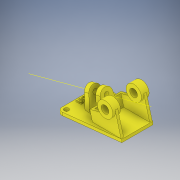
# Autodesk Inventor part: Piesa 1
Saved by Autodesk Inventor 2019.4 (Build 234330000, 330)
## iProperties
Created: 2020-02-23
Part Number: Piesa 1
Material: Steel, Carbon
Document SubType Name: Modeling
Designer: Gabriel
Density: 7.85 g/cm^3
Appearance: Canary
Author: Gabriel
Autodesk Inventor part; units mm, degrees
ref_plane "YZ Plane" through (0, 0, 0) normal (1, 0, 0) x (0, 1, 0)
ref_plane "XZ Plane" through (0, 0, 0) normal (0, 1, 0) x (-1, 0, 0)
ref_plane "XY Plane" through (0, 0, 0) normal (0, 0, 1) x (1, 0, 0)
sketch "Sketch1" plane through (0, 0, 0) normal (0, 0, 1) x (1, 0, 0)
  line L0 (-28.987733, 0) -> (173.926398, 0)
  line L1 (176.623272, 47.326063) -> (-29.437212, -7.887677)
  line L2 (101.214161, 39.543567) -> (109.907493, 41.872938)
  line L3 (109.907493, 41.872938) -> (118.96616, 8.065534)
  line L4 (118.96616, 8.065534) -> (132.489121, 11.689001)
  line L5 (132.489121, 11.689001) -> (123.430455, 45.496405)
  line L6 (123.430455, 45.496405) -> (132.123787, 47.825776)
  line L7 (132.123787, 47.825776) -> (144.938665, 0)
  line L8 (144.938665, 0) -> (111.809827, 0)
  line L9 (111.809827, 0) -> (101.214161, 39.543567)
  point P0 (0, 0)
  dimension "d0" = 9
  dimension "d1" = 14
  dimension "d2" = 9
  dimension "d3" = 35
  dimension "d4" = 117
  dimension "d5" = 12
  constraints: 16 end point, 6 perpendicular, 1 collinear, 1 horizontal, 1 point on line
  measures "d0" distance of L2.start L2.end
  measures "d1" distance of L3.end L4.end
  measures "d2" distance of L5.end L6.end
  measures "d3" distance between parallel lines of L2 L4
  measures "d4" distance from line of point (0, 0) L3
  measures "d5" distance between parallel lines of L6 L1
extrude "Extrusion1" add sketch "Sketch1" along normal mid plane 50 contours L9 L1 L3 L4 L5 L7 L0 | L9 L2 L3 L1 | L1 L5 L6 L7
sketch "Sketch2" plane through (111.809827, 0, -25) normal (-0.9659258, -0.258819, 0) x (0, 0, 1)
  line L0 (25, 64.840128) -> (25, -46.47118)
  line L1 (50, -8.574374) -> (0, -8.574374)
  line L2 (0, 40.938513) -> (50, 40.938513)
  line L3 (1.569954, -23.574374) -> (48.430046, -23.574374)
  line L4 (48.430046, -23.574374) -> (36.737771, 31.433453)
  line L5 (1.569954, -23.574374) -> (13.262229, 31.433453)
  arc A0 (36.737771, 31.433453) -> (13.262229, 31.433453) centre (25, 28.938513) ccw
  point P0 (25, 28.938513)
  point P1 (25, 40.938513)
  dimension "d8" = 15
  dimension "d9" = 12
  dimension "d10" = 78
  dimension "d11" = 78
  constraints: 6 end point, 3 point on circle, 2 tangent, 1 centre point, 1 horizontal, 1 midpoint
  measures "d8" distance between parallel lines of L1 L3
  measures "d9" radius of A0
  measures "d10" angle of L5 L3
  measures "d11" angle of L3 L4
extrude "Extrusion2" cut sketch "Sketch2" against normal through all keep common part
sketch "Sketch3" plane through (0, 0, 0) normal (0, 0, 1) x (1, 0, 0)
  line L0 (176.623272, 47.326063) -> (-29.437212, -7.887677)
  line L1 (-28.987733, 0) -> (173.926398, 0)
  line L2 (132.98317, 25.3) -> (156.16539, 31.511657)
  line L3 (156.16539, 31.511657) -> (153.582206, 41.152228)
  line L4 (182.559981, 48.9168) -> (195.667198, 0)
  line L5 (195.667198, 0) -> (139.762284, 0)
  line L6 (132.98317, 25.3) -> (139.762284, 0)
  point P0 (0, 0)
  point P1 (144.938665, 0)
  dimension "d14" = 24
  dimension "d15" = 30
  dimension "d16" = 49
  dimension "d17" = 5
  dimension "d18" = 25.3
  constraints: 10 end point, 4 point on line, 2 perpendicular, 1 parallel
  measures "d14" distance of L2.start L2.end
  measures "d15" distance between parallel lines of L4 L3
  measures "d16" distance from line of point (144.939, 0) L4
  measures "d17" distance from line of point (144.939, 0) L6
  measures "d18" distance from line of L1 L2.start
sketch "Sketch3 outline for Extrusion3" plane through (0, 0, 0) normal (0, 0, 1) x (1, 0, 0)
  line L0 (156.16539, 31.511657) -> (132.98317, 25.3)
  line L1 (153.582206, 41.152228) -> (156.16539, 31.511657)
  line L2 (182.559981, 48.9168) -> (153.582206, 41.152228)
  line L3 (195.667198, 0) -> (182.559981, 48.9168)
  line L4 (139.762284, 0) -> (195.667198, 0)
  line L5 (132.98317, 25.3) -> (139.762284, 0)
extrude "Extrusion3" add sketch "Sketch3 outline for Extrusion3" along normal mid plane 61
sketch "Sketch4" plane through (153.582206, 41.152228, 30.5) normal (-0.258819, 0.9659258, 0) x (0.9659258, 0.258819, 0)
  line L0 (35, 56) -> (5, 56)
  line L1 (5, 56) -> (5, 5)
  line L2 (5, 5) -> (35, 5)
  line L3 (35, 5) -> (35, 56)
  line L4 (0, 61) -> (30, 61) projected
  line L5 (30, 0) -> (0, 0) projected
  line L6 (30, 61) -> (30, 0) projected
  line L7 (0, 61) -> (0, 0) projected
  point P0 (-159, 30.5)
  dimension "d21" = 5
  dimension "d22" = 5
  dimension "d23" = 5
  dimension "d24" = 5
  constraints: 8 end point, 2 parallel, 1 horizontal, 1 perpendicular
  measures "d21" distance between parallel lines of L0 L4
  measures "d22" distance between parallel lines of L5 L2
  measures "d23" distance between parallel lines of L6 L3
  measures "d24" distance between parallel lines of L1 L7
extrude "Extrusion4" cut sketch "Sketch4" against normal through all contours L3 L2 L6 L0 | L6 L2 L1 L0
sketch "Sketch5" plane through (156.16539, 31.511657, 30.5) normal (-0.258819, 0.9659258, 0) x (0.9659258, 0.258819, 0)
  line L0 (32.064075, 5) -> (-19, 5)
  line L1 (-19, 5) -> (-19, 56)
  line L2 (-19, 56) -> (32.064075, 56)
  line L3 (32.064075, 56) -> (32.064075, 5)
  line L4 (-24, 61) -> (0, 61)
  line L5 (5, 56) -> (30, 56)
  line L6 (-19, 16.110459) -> (-19, 44.889541)
  line L7 (30, 5) -> (5, 5)
  point P0 (-159, 30.5)
  constraints: 8 end point, 3 collinear, 3 parallel, 1 horizontal, 1 perpendicular
extrude "Extrusion5" cut sketch "Sketch5" along normal through all both and the other way through all
sketch "Sketch6" plane through (0, 0, 0) normal (0, 0, 1) x (1, 0, 0)
  line L0 (153.582206, 41.152228) -> (182.559981, 48.9168)
  circle A0 centre (168.071094, 45.034514) radius 15
  point P0 (0, 0)
  constraints: 1 midpoint, 3 other
extrude "Extrusion6" add sketch "Sketch6" along normal mid plane 71
sketch "Sketch7" plane through (0, 0, 0) normal (0, 0, 1) x (1, 0, 0)
  circle A0 centre (168.071094, 45.034514) radius 15
  circle A1 centre (168.071094, 45.034514) radius 19.5
  point P0 (0, 0)
  dimension "d31" = 39
  constraints: 1 centre point, 1 coincident
  measures "d31" diameter of A1
extrude "Extrusion7" cut sketch "Sketch7" along normal mid plane 41
sketch "Sketch8" plane through (0, 0, 0) normal (0, 0, 1) x (1, 0, 0)
  circle A0 centre (168.071094, 45.034514) radius 15
  circle A1 centre (168.071094, 45.034514) radius 15
  point P0 (0, 0)
  dimension "d34" = 30
  constraints: 1 centre point, 1 coincident
  measures "d34" diameter of A1
extrude "Extrusion8" cut sketch "Sketch8" along normal mid plane 41
sketch "Sketch9" plane through (111.809827, 0, -18.419158) normal (0, -1, 0) x (1, 0, 0)
  line L0 (83.857371, -12.080842) -> (83.857371, 48.919158)
  line L1 (83.857371, 48.919158) -> (-20.192674, 61.362557)
  line L2 (-29.142629, 53.419158) -> (-29.142629, -16.580842)
  line L3 (-20.192674, -24.524241) -> (83.857371, -12.080842)
  line L4 (70.750154, -12.080842) -> (83.857371, -12.080842)
  arc A0 (-29.142629, -16.580842) -> (-20.192674, -24.524241) centre (-21.142629, -16.580842) ccw
  arc A1 (-20.192674, 61.362557) -> (-29.142629, 53.419158) centre (-21.142629, 53.419158) ccw
  line L5 (122.99081, 18.419158) -> (-150.943267, 18.419158)
  point P0 (-111.809827, 18.419158)
  dimension "d37" = 8
  dimension "d38" = 70
  dimension "d39" = 113
  dimension "d40" = 35
  constraints: 8 end point, 4 point on circle, 4 tangent, 2 centre point, 2 vertical, 1 coincident, 1 equal radius, 1 point on line
  measures "d37" radius of A0
  measures "d38" distance of A1.centre A0.centre
  measures "d39" distance between parallel lines of L2 L0
  measures "d40" distance from line of L5 A0.centre
extrude "Extrusion9" add sketch "Sketch9" against normal blind 6
sketch "Sketch10" plane through (168.071094, 45.034514, 35.5) normal (0, 0, 1) x (1, 0, 0)
  point P0 (-168.071094, -45.034514)
  point P1 (-0.346421, -0.168728)
hole "Hole1" at (167.724672, 44.865786, 35.5) direction (0, 0, -1) diameter 15 end through all
hole "Hole2" at (96.592583, 25.881905, 0) direction (0.9659258, 0.258819, 0) diameter 9 end through all
sketch "Sketch11" plane through (111.809827, 6, -18.419158) normal (0, 1, 0) x (1, 0, 0)
  line L0 (83.857371, 12.080842) -> (-20.192674, 24.524241)
  line L1 (-29.142629, 16.580842) -> (-29.142629, -53.419158)
  point P0 (-111.809827, -18.419158)
  point P1 (-20.642629, 16.017484)
  dimension "d59" = 8.5
  dimension "d60" = 8.5
  measures "d59" distance from line of L0 point (-20.643, 16.017)
  measures "d60" distance from line of L1 point (-20.643, 16.017)
hole "Hole3" at (91.167198, 6, -34.436642) direction (0, -1, 0) diameter 9 end through all
sketch "Sketch12" plane through (111.809827, 6, -18.419158) normal (0, 1, 0) x (1, 0, 0)
  line L0 (-20.192674, -61.362557) -> (83.857371, -48.919158)
  line L1 (-29.142629, 16.580842) -> (-29.142629, -53.419158)
  point P0 (-111.809827, -18.419158)
  point P1 (-20.642629, -52.8558)
  dimension "d68" = 8.5
  dimension "d69" = 8.5
  measures "d68" distance from line of L0 point (-20.643, -52.856)
  measures "d69" distance from line of L1 point (-20.643, -52.856)
hole "Hole4" at (91.167198, 6, 34.436642) direction (0, -1, 0) diameter 9 end through all
sketch "Sketch13" plane through (111.809827, 6, -18.419158) normal (0, 1, 0) x (1, 0, 0)
  line L0 (-25.142629, -32.919158) -> (-25.142629, -3.919158) construction
  line L1 (-25.142629, -3.919158) -> (-14.142629, -3.919158) construction
  line L2 (-14.142629, -3.919158) -> (-14.142629, -32.919158) construction
  line L3 (-14.142629, -32.919158) -> (-25.142629, -32.919158) construction
  line L4 (-29.142629, 16.580842) -> (-29.142629, -53.419158)
  line L5 (122.99081, -18.419158) -> (-150.943267, -18.419158)
  spline S0 degree 2 poles (-14.44814, -26.713323) (-14.44814, -27.596629) (-14.910052, -28.909433) (-15.371965, -29.371346) knots 0 0 0 1 2 2 2
  spline S1 degree 2 poles (-15.371965, -29.371346) (-15.890603, -29.898088) (-17.349274, -30.327585) (-18.418966, -30.327585) knots 0 0 0 1 2 2 2
  line L6 (-18.418966, -30.327585) -> (-24.658837, -30.327585)
  line L7 (-24.658837, -30.327585) -> (-24.658837, -28.998574)
  line L8 (-24.658837, -28.998574) -> (-18.418966, -28.998574)
  spline S2 degree 2 poles (-18.418966, -28.998574) (-17.722046, -28.998574) (-16.782013, -28.820292) (-16.401138, -28.569077) knots 0 0 0 1 2 2 2
  spline S3 degree 2 poles (-16.401138, -28.569077) (-15.995952, -28.301654) (-15.582662, -27.377829) (-15.582662, -26.713323) knots 0 0 0 1 2 2 2
  spline S4 degree 2 poles (-15.582662, -26.713323) (-15.582662, -26.089336) (-15.995952, -25.116889) (-16.401138, -24.849466) knots 0 0 0 1 2 2 2
  spline S5 degree 2 poles (-16.401138, -24.849466) (-16.782013, -24.59825) (-17.713942, -24.419968) (-18.386551, -24.419968) knots 0 0 0 1 2 2 2
  line L9 (-18.386551, -24.419968) -> (-24.658837, -24.419968)
  line L10 (-24.658837, -24.419968) -> (-24.658837, -23.090957)
  line L11 (-24.658837, -23.090957) -> (-18.418966, -23.090957)
  spline S6 degree 2 poles (-18.418966, -23.090957) (-17.373586, -23.090957) (-15.8825, -23.51235) (-15.371965, -24.047196) knots 0 0 0 1 2 2 2
  spline S7 degree 2 poles (-15.371965, -24.047196) (-14.901949, -24.525316) (-14.44814, -25.789498) (-14.44814, -26.713323) knots 0 0 0 1 2 2 2
  spline S8 degree 2 poles (-14.480555, -17.280584) (-14.480555, -18.253031) (-15.136957, -19.898088) (-15.793359, -20.497764) knots 0 0 0 1 2 2 2
  spline S9 degree 2 poles (-15.793359, -20.497764) (-16.441657, -21.09744) (-18.386551, -21.753842) (-19.650733, -21.753842) knots 0 0 0 1 2 2 2
  spline S10 degree 2 poles (-19.650733, -21.753842) (-20.906811, -21.753842) (-22.770668, -21.113647) (-23.459485, -20.505867) knots 0 0 0 1 2 2 2
  spline S11 degree 2 poles (-23.459485, -20.505867) (-24.132094, -19.906192) (-24.837119, -18.269239) (-24.837119, -17.256273) knots 0 0 0 1 2 2 2
  spline S12 degree 2 poles (-24.837119, -17.256273) (-24.837119, -16.753842) (-24.691252, -15.870535) (-24.577799, -15.497764) knots 0 0 0 1 2 2 2
  spline S13 degree 2 poles (-24.577799, -15.497764) (-24.472451, -15.173615) (-24.172613, -14.501005) (-23.994331, -14.168752) knots 0 0 0 1 2 2 2
  line L12 (-23.994331, -14.168752) -> (-22.389793, -14.168752)
  line L13 (-22.389793, -14.168752) -> (-22.389793, -14.274101)
  spline S14 degree 2 poles (-22.389793, -14.274101) (-22.551868, -14.452383) (-23.005676, -15.003436) (-23.224477, -15.400519) knots 0 0 0 1 2 2 2
  spline S15 degree 2 poles (-23.224477, -15.400519) (-23.435174, -15.781394) (-23.702597, -16.680908) (-23.702597, -17.264376) knots 0 0 0 1 2 2 2
  spline S16 degree 2 poles (-23.702597, -17.264376) (-23.702597, -17.904571) (-23.175855, -19.047196) (-22.673423, -19.476694) knots 0 0 0 1 2 2 2
  spline S17 degree 2 poles (-22.673423, -19.476694) (-22.162889, -19.898088) (-20.615077, -20.368104) (-19.650733, -20.368104) knots 0 0 0 1 2 2 2
  spline S18 degree 2 poles (-19.650733, -20.368104) (-18.62156, -20.368104) (-17.138577, -19.873777) (-16.628043, -19.444279) knots 0 0 0 1 2 2 2
  spline S19 degree 2 poles (-16.628043, -19.444279) (-16.133715, -19.022885) (-15.631284, -17.896467) (-15.631284, -17.264376) knots 0 0 0 1 2 2 2
  spline S20 degree 2 poles (-15.631284, -17.264376) (-15.631284, -16.689012) (-15.914915, -15.708461) (-16.125611, -15.327585) knots 0 0 0 1 2 2 2
  spline S21 degree 2 poles (-16.125611, -15.327585) (-16.336308, -14.962918) (-16.77391, -14.419968) (-16.92788, -14.265997) knots 0 0 0 1 2 2 2
  line L14 (-16.92788, -14.265997) -> (-16.92788, -14.168752)
  line L15 (-16.92788, -14.168752) -> (-15.33955, -14.168752)
  spline S22 degree 2 poles (-15.33955, -14.168752) (-15.185579, -14.501005) (-14.901949, -15.084474) (-14.772289, -15.497764) knots 0 0 0 1 2 2 2
  spline S23 degree 2 poles (-14.772289, -15.497764) (-14.626422, -15.935365) (-14.480555, -16.680908) (-14.480555, -17.280584) knots 0 0 0 1 2 2 2
  line L16 (-24.658837, -5.676046) -> (-14.658837, -9.12013)
  line L17 (-14.658837, -9.12013) -> (-14.658837, -10.55449)
  line L18 (-14.658837, -10.55449) -> (-24.658837, -13.998574)
  line L19 (-24.658837, -13.998574) -> (-24.658837, -12.572318)
  line L20 (-24.658837, -12.572318) -> (-16.352516, -9.800843)
  line L21 (-16.352516, -9.800843) -> (-24.658837, -7.029368)
  line L22 (-24.658837, -7.029368) -> (-24.658837, -5.676046)
  point P0 (-111.809827, -18.419158)
  dimension "d77" = 4
  dimension "d78" = 11
  dimension "d79" = 29
  dimension "d80" = 14.5
  constraints: 1 parallel, 2 other
  measures "d77" distance between parallel lines of L4 L0
  measures "d78" distance between parallel lines of L2 L0
  measures "d79" distance between parallel lines of L1 L3
  measures "d80" distance between parallel lines of L5 L3
emboss "Emboss1" sketch "Sketch13" operation add depth 2 direction (0, -1, 0) contours S8 S9 S10 S11 L5 S16 S17 S18 S19 | L5 S19 S20 S21 L14 L15 S22 S23 S8 | L5 S11 S12 S13 L12 L13 S14 S15 S16 | S0 S1 L6 L7 L8 S2 S3 S4 S5 L9 L10 L11 S6 S7 | L16 L17 L18 L19 L20 L21 L22
body "Solid1"
